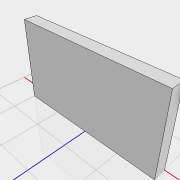
# Autodesk Inventor part: ЛЦМК000002.00.00.00.00.17
Saved by Autodesk Inventor 2021.2 (Build 252289000, 289)
## iProperties
Created: 2025-11-09
Part Number: ЛЦМК000002.00.00.00.00.17
Material: Типовые
Document SubType Name: Modeling
Designer: Захаров
Density: 1 g/cm^3
Appearance: По умолчанию
Author: Захаров
Autodesk Inventor part; units mm, degrees
ref_plane "YZ Plane" through (0, 0, 0) normal (1, 0, 0) x (0, 1, 0)
ref_plane "XZ Plane" through (0, 0, 0) normal (0, 1, 0) x (-1, 0, 0)
ref_plane "XY Plane" through (0, 0, 0) normal (0, 0, 1) x (1, 0, 0)
sketch "Эскиз1" plane through (0, 0, 0) normal (0, 0, 1) x (1, 0, 0)
  line L0 (-40, 22.25) -> (40, 22.25)
  line L1 (40, 22.25) -> (40, -22.25)
  line L2 (40, -22.25) -> (-40, -22.25)
  line L3 (-40, -22.25) -> (-40, 22.25)
  line L4 (-40, 22.25) -> (40, -22.25) construction
  line L5 (40, 22.25) -> (-40, -22.25) construction
  point P0 (0, 0)
  dimension "d0" = 80
  dimension "d1" = 44.5
  constraints: 12 end point, 2 midpoint, 2 parallel, 1 horizontal, 1 perpendicular
  measures "d0" distance of L1.end L2.end
  measures "d1" distance of L0.end L1.end
extrude "Выдавливание1" add sketch "Эскиз1" along normal blind 7
